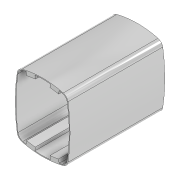
# Autodesk Inventor part: lineaire as deel 2
Saved by Autodesk Inventor 2020.3 (Build 243373000, 373)
## iProperties
Created: 2020-09-16
Part Number: lineaire as deel 2
Material: Aluminum 6061
Document SubType Name: Modeling
Designer: Svend
Density: 2.7 g/cm^3
Appearance: Aluminum - Polished
Author: Svend
Autodesk Inventor part; units mm, degrees
ref_plane "YZ Plane" through (0, 0, 0) normal (1, 0, 0) x (0, 1, 0)
ref_plane "XZ Plane" through (0, 0, 0) normal (0, 1, 0) x (-1, 0, 0)
ref_plane "XY Plane" through (0, 0, 0) normal (0, 0, 1) x (1, 0, 0)
sketch "Sketch1" plane through (0, 0, 0) normal (0, 0, 1) x (1, 0, 0)
  line L0 (-57, -57.5) -> (57, 57.5) construction
  line L1 (-67.5, 67.5) -> (67.5, 67.5) construction
  line L2 (67.5, 67.5) -> (67.5, -67.5) construction
  line L3 (67.5, -67.5) -> (-67.5, -67.5) construction
  line L4 (-67.5, -67.5) -> (-67.5, 67.5) construction
  line L5 (-67.5, 67.5) -> (67.5, -67.5) construction
  line L6 (67.5, 67.5) -> (-67.5, -67.5) construction
  circle A0 centre (-37.5, 37.5) radius 4
  circle A1 centre (-37.5, -37.5) radius 4
  circle A2 centre (37.5, -37.5) radius 4
  circle A3 centre (37.5, 37.5) radius 4
  arc A4 (-48.5, 62.5) -> (-48.5, -62.5) centre (326.325, 0) ccw
  line L7 (0, 67.5) -> (0, -67.5) construction
  line L8 (67.5, -67.5) -> (67.5, 67.5) construction
  arc A5 (48.5, -62.5) -> (48.5, 62.5) centre (-326.325, 0) ccw
  arc A6 (48.5, 62.5) -> (-48.5, 62.5) centre (0, -110.8429) ccw
  line L9 (-67.5, 0) -> (53.675, 0) construction
  arc A7 (-48.5, -62.5) -> (48.5, -62.5) centre (0, 110.8429) ccw
  arc A8 (-30.7003, 46.1842) -> (-30.7003, -46.1842) centre (326.325, 0) ccw
  arc A9 (-30.7003, -46.1842) -> (30.7003, -46.1842) centre (0, 110.8429) ccw
  arc A10 (30.7003, -46.1842) -> (30.7003, 46.1842) centre (-326.325, 0) ccw
  arc A11 (30.7003, 46.1842) -> (-30.7003, 46.1842) centre (0, -110.8429) ccw
  arc A12 (-55.5322, 68.7683) -> (-55.5322, -68.7683) centre (326.325, 0) ccw
  arc A13 (-55.5322, -68.7683) -> (55.5322, -68.7683) centre (0, 110.8429) ccw
  arc A14 (55.5322, -68.7683) -> (55.5322, 68.7683) centre (-326.325, 0) ccw
  arc A15 (55.5322, 68.7683) -> (-55.5322, 68.7683) centre (0, -110.8429) ccw
  arc A16 (-57.2838, 70.3161) -> (-57.2838, -70.3161) centre (326.325, 0) ccw
  arc A17 (-57.2838, -70.3161) -> (57.2838, -70.3161) centre (0, 110.8429) ccw
  arc A18 (57.2838, -70.3161) -> (57.2838, 70.3161) centre (-326.325, 0) ccw
  arc A19 (57.2838, 70.3161) -> (-57.2838, 70.3161) centre (0, -110.8429) ccw
  line L10 (17.7854, 76.314) -> (17.0881, 68.3442)
  line L11 (38.478, 73.1774) -> (37.0881, 65.2948)
  line L12 (-17.7854, 76.314) -> (-17.0881, 68.3442)
  line L13 (-38.478, 73.1774) -> (-37.0881, 65.2948)
  line L14 (17.7854, -76.314) -> (17.0881, -68.3442)
  line L15 (38.478, -73.1774) -> (37.0881, -65.2948)
  line L16 (-38.478, -73.1774) -> (-37.0881, -65.2948)
  line L17 (-17.7854, -76.314) -> (-17.0881, -68.3442)
  point P0 (0, 0)
  point P1 (0, 0)
  point P2 (-53.675, 0)
  point P3 (0, 0)
  dimension "d3" = 135
  dimension "d4" = 135
  dimension "d5" = 8
  dimension "d9" = 360
  dimension "d29" = 75
  dimension "d30" = 125
  dimension "d31" = 97
  dimension "d32" = 180
  dimension "d33" = 380
  dimension "d34" = 20
  dimension "d36" = 8
  dimension "d37" = 2
  dimension "d38" = 5
  dimension "d39" = 20
  dimension "d41" = 5
  constraints: 37 point on circle, 36 end point, 20 centre point, 17 symmetric about line, 7 midpoint, 2 horizontal, 2 parallel, 1 coincident, 1 horizontal alignment, 1 perpendicular, 1 point on line, 20 other
  measures "d3" distance of L2.end L3.end
  measures "d4" distance of L1.end L2.end
  measures "d5" diameter of A0
  measures "d29" distance of A0.centre A3.centre
  measures "d30" distance of A4.end A4.start
  measures "d31" distance of A5.end A4.start
  measures "d32" radius of A6
  measures "d33" radius of A4
  measures "d34" radial gap between concentric circles of A6 A11
  measures "d36" radial gap between concentric circles of A6 A15
  measures "d37" radial gap between concentric circles of A15 A19
  measures "d38" angle of L10 L11
  measures "d39" horizontal distance of L10.end L11.end
  measures "d41" angle of L7 L10
extrude "Extrusion1" add sketch "Sketch1" along normal mid plane 220 contours L13 A15 L12 A6 | A7 L17 A13 L16 | L10 A15 L11 A6 | A7 L15 A13 L14 | A19 A18 A17 A16
fillet "Fillet2" radius 15 8 edges at (57.2838, 70.3161, 0) (-57.2838, 70.3161, 0) (-57.2838, -70.3161, 0) (57.2838, -70.3161, 0) (55.5322, -68.7683, 0) (-55.5322, -68.7683, 0) (-55.5322, 68.7683, 0) (55.5322, 68.7683, 0)
body "Solid1"
